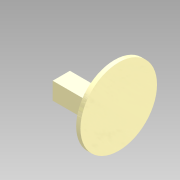
# Autodesk Inventor part: propellor_fuselage_interface
Saved by Autodesk Inventor 2021 (Build 250183000, 183)
## iProperties
Created: 2020-11-15
Part Number: propellor_fuselage_interface
Material: Nylon 6/6
Document SubType Name: Modeling
Designer: Paco
Density: 1.13 g/cm^3
Appearance: Nylon 6
Mass: 3.1027 g
Surface Area: 36.8195 cm^2
Volume: 2.74575 cm^3
Author: Paco
Autodesk Inventor part; units mm, degrees
ref_plane "YZ Plane" through (0, 0, 0) normal (1, 0, 0) x (0, 1, 0)
ref_plane "XZ Plane" through (0, 0, 0) normal (0, 1, 0) x (-1, 0, 0)
ref_plane "XY Plane" through (0, 0, 0) normal (0, 0, 1) x (1, 0, 0)
sketch "Sketch3" plane through (0, 0, 0) normal (1, 0, 0) x (0, 1, 0)
  line L0 (3.05, -3.05) -> (-3.05, -3.05)
  line L1 (-3.05, -3.05) -> (-3.05, 3.05)
  line L2 (-3.05, 3.05) -> (3.05, 3.05)
  line L3 (3.05, 3.05) -> (3.05, -3.05)
  line L4 (3.05, -3.05) -> (-3.05, 3.05) construction
  line L5 (-3.05, -3.05) -> (3.05, 3.05) construction
  line L6 (4.05, -4.05) -> (-4.05, -4.05)
  line L7 (-4.05, -4.05) -> (-4.05, 4.05)
  line L8 (-4.05, 4.05) -> (4.05, 4.05)
  line L9 (4.05, 4.05) -> (4.05, -4.05)
  line L10 (4.05, -4.05) -> (-4.05, 4.05) construction
  line L11 (-4.05, -4.05) -> (4.05, 4.05) construction
  point P0 (0, 0)
  point P1 (0, 0)
  point P2 (0, 0)
  dimension "d38" = 8.1
  dimension "d39" = 8.1
  dimension "d40" = 6.1
  dimension "d41" = 6.1
  constraints: 24 end point, 5 midpoint, 4 parallel, 2 horizontal, 2 perpendicular, 1 coincident, 1 point on line, 1 other
  measures "d38" distance of L8.end L6.start
  measures "d39" distance of L7.end L8.end
  measures "d40" distance of L2.end L0.start
  measures "d41" distance of L1.end L2.end
extrude "Extrusion2" add sketch "Sketch3" along normal blind 25
sketch "Sketch9" plane through (25, 0, 0) normal (1, 0, 0) x (0, 0, -1)
  line L0 (-4.05, 4.05) -> (-4.05, -4.05) projected
  line L1 (-4.05, -4.05) -> (4.05, -4.05) projected
  line L2 (4.05, -4.05) -> (4.05, 4.05) projected
  line L3 (4.05, 4.05) -> (-4.05, 4.05) projected
  line L4 (3.05, 3.05) -> (3.05, -3.05) projected
  line L5 (3.05, -3.05) -> (-3.05, -3.05) projected
  line L6 (-3.05, -3.05) -> (-3.05, 3.05) projected
  line L7 (-3.05, 3.05) -> (3.05, 3.05) projected
  circle A0 centre (0, 5) radius 18
  line L8 (0, 0) -> (0, 9.371) construction
  dimension "d42" = 5
  dimension "d45" = 36
  constraints: 2 end point, 1 centre point, 1 point on line, 1 vertical
  measures "d42" distance of A0.centre L8.start
  measures "d45" diameter of A0
extrude "Extrusion6" add sketch "Sketch9" along normal blind 2 contours L3 L2 L1 L0 | L4 L5 L6 L7 | A0
equation "\"d39\" = d38"
body "Solid2"
